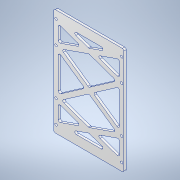
# Autodesk Inventor part: 関節2_上板
Saved by Autodesk Inventor 2021 (Build 250183000, 183)
## iProperties
Created: 2022-02-02
Part Number: 関節2_上板
Material: アルミニウム 6061
Document SubType Name: Modeling
Designer: hirohumi
Density: 2.7 g/cm^3
Appearance: アルミニウム - フラット
Mass: 103.807 g
Surface Area: 272.646 cm^2
Volume: 38.447 cm^3
Author: hirohumi
Autodesk Inventor part; units mm, degrees
ref_plane "YZ Plane" through (0, 0, 0) normal (1, 0, 0) x (0, 1, 0)
ref_plane "XZ Plane" through (0, 0, 0) normal (0, 1, 0) x (-1, 0, 0)
ref_plane "XY Plane" through (0, 0, 0) normal (0, 0, 1) x (1, 0, 0)
sketch "スケッチ1" plane through (0, 0, 0) normal (0, 0, 1) x (1, 0, 0)
  line L0 (46, 70) -> (-46, 70)
  line L1 (-46, 70) -> (-46, -70)
  line L2 (-46, -70) -> (46, -70)
  line L3 (46, -70) -> (46, 70)
  line L4 (46, 70) -> (-46, -70) construction
  line L5 (-46, 70) -> (46, -70) construction
  circle A0 centre (-43, 60) radius 1.6
  circle A1 centre (-43, 30) radius 1.6
  circle A2 centre (-43, -30) radius 1.6
  circle A3 centre (-43, -60) radius 1.6
  circle A4 centre (43, 60) radius 1.6
  circle A5 centre (43, 30) radius 1.6
  circle A6 centre (43, -30) radius 1.6
  circle A7 centre (43, -60) radius 1.6
  point P0 (0, 0)
  dimension "d0" = 92
  dimension "d1" = 140
  dimension "d2" = 3.2
  dimension "d3" = 3.2
  dimension "d4" = 3.2
  dimension "d5" = 3.2
  dimension "d6" = 120
  dimension "d7" = 10
  dimension "d8" = 30
  dimension "d9" = 30
  dimension "d10" = 3.2
  dimension "d11" = 3.2
  dimension "d12" = 3.2
  dimension "d13" = 3.2
  dimension "d14" = 120
  dimension "d15" = 30
  dimension "d16" = 30
  dimension "d17" = 3
  dimension "d18" = 3
  dimension "d19" = 60
  constraints: 12 end point, 8 centre point, 6 vertical alignment, 2 midpoint, 2 parallel, 1 horizontal, 1 perpendicular
  measures "d0" distance of L2.end L1.end
  measures "d1" distance of L1.end L0.end
  measures "d2" diameter of A0
  measures "d3" diameter of A1
  measures "d4" diameter of A2
  measures "d5" diameter of A3
  measures "d6" distance of A3.centre A0.centre
  measures "d7" distance from line of L0 A0.centre
  measures "d8" distance of A1.centre A0.centre
  measures "d9" distance of A3.centre A2.centre
  measures "d10" diameter of A4
  measures "d11" diameter of A5
  measures "d12" diameter of A6
  measures "d13" diameter of A7
  measures "d14" distance of A7.centre A4.centre
  measures "d15" distance of A5.centre A4.centre
  measures "d16" distance of A7.centre A6.centre
  measures "d17" distance from line of L1 A1.centre
  measures "d18" distance from line of L3 A5.centre
  measures "d19" vertical distance of point (0, 0) A4.centre
extrude "押し出し1" add sketch "スケッチ1" along normal blind 3
fillet "フィレット1" radius 2 4 edges at (-46, 70, 1.5) (46, 70, 1.5) (-46, -70, 1.5) (46, -70, 1.5)
sketch "スケッチ2" plane through (0, 0, 3) normal (0, 0, 1) x (1, 0, 0)
  circle A0 centre (-43, 60) radius 1.6 projected
  circle A1 centre (43, 30) radius 1.6 projected
  line L0 (-43, 60) -> (43, 30) construction
  circle A2 centre (-43, 30) radius 1.6 projected
  circle A3 centre (43, -30) radius 1.6 projected
  line L1 (-43, 30) -> (43, -30) construction
  circle A4 centre (-43, -60) radius 1.6 projected
  line L2 (43, -30) -> (-43, -60) construction
  circle A5 centre (43, -60) radius 1.6 projected
  line L3 (-43, -60) -> (43, -60) construction
  circle A6 centre (-43, -30) radius 1.6 projected
  line L4 (43, -60) -> (-43, -30) construction
  line L5 (-43, -30) -> (43, 30) construction
  circle A7 centre (43, 60) radius 1.6 projected
  line L6 (-43, 60) -> (43, 60) construction
  line L7 (43, 60) -> (-43, 30) construction
  line L8 (-43, 60) -> (-43, -60) construction
  line L9 (43, 60) -> (43, -60) construction
  line L10 (-40, 55.7762) -> (-40, 34.2238)
  line L11 (-40, 34.2238) -> (-9.1082, 45)
  line L12 (-9.1082, 45) -> (-40, 55.7762)
  line L13 (9.1082, 45) -> (40, 34.2238)
  line L14 (40, 34.2238) -> (40, 55.7762)
  line L15 (40, 55.7762) -> (9.1082, 45)
  line L16 (-28.1584, 58) -> (0, 48.1773)
  line L17 (0, 48.1773) -> (28.1584, 58)
  line L18 (28.1584, 58) -> (-28.1584, 58)
  line L19 (-36.4685, 29.1011) -> (0, 41.8227)
  line L20 (0, 41.8227) -> (36.4685, 29.1011)
  line L21 (36.4685, 29.1011) -> (0, 3.658)
  line L22 (0, 3.658) -> (-36.4685, 29.1011)
  line L23 (-40, 24.249) -> (-40, -24.249)
  line L24 (-40, -24.249) -> (-5.2431, 0)
  line L25 (-5.2431, 0) -> (-40, 24.249)
  line L26 (5.2431, 0) -> (40, -24.249)
  line L27 (40, -24.249) -> (40, 24.249)
  line L28 (5.2431, 0) -> (40, 24.249)
  line L29 (-36.4685, -29.1011) -> (0, -41.8227)
  line L30 (0, -41.8227) -> (36.4685, -29.1011)
  line L31 (36.4685, -29.1011) -> (0, -3.658)
  line L32 (0, -3.658) -> (-36.4685, -29.1011)
  line L33 (-40, -34.2238) -> (-40, -55.7762)
  line L34 (-40, -55.7762) -> (-9.1082, -45)
  line L35 (-9.1082, -45) -> (-40, -34.2238)
  line L36 (9.1082, -45) -> (40, -55.7762)
  line L37 (40, -55.7762) -> (40, -34.2238)
  line L38 (40, -34.2238) -> (9.1082, -45)
  line L39 (0, -48.1773) -> (-28.1584, -58)
  line L40 (-28.1584, -58) -> (28.1584, -58)
  line L41 (28.1584, -58) -> (0, -48.1773)
  point P0 (0, 0)
  dimension "d23" = 2
  dimension "d24" = 3
  dimension "d25" = 3
  dimension "d26" = 3
  dimension "d27" = 3
  dimension "d28" = 3
  dimension "d29" = 3
  dimension "d30" = 3
  dimension "d31" = 3
  dimension "d32" = 3
  dimension "d33" = 3
  dimension "d34" = 3
  dimension "d35" = 3
  dimension "d36" = 3
  dimension "d37" = 3
  dimension "d38" = 3
  dimension "d39" = 3
  dimension "d40" = 3
  dimension "d41" = 3
  dimension "d42" = 3
  dimension "d43" = 3
  dimension "d44" = 3
  dimension "d45" = 3
  dimension "d46" = 3
  dimension "d47" = 3
  dimension "d48" = 3
  dimension "d49" = 3
  dimension "d50" = 3
  dimension "d51" = 3
  dimension "d52" = 2
  constraints: 84 end point, 33 parallel, 2 point on line, 1 collinear, 1 horizontal, 1 vertical
  measures "d23" distance between parallel lines of L6 L18
  measures "d24" distance between parallel lines of L0 L16
  measures "d25" distance between parallel lines of L7 L17
  measures "d26" distance between parallel lines of L0 L12
  measures "d27" distance between parallel lines of L7 L15
  measures "d28" distance between parallel lines of L9 L14
  measures "d29" distance between parallel lines of L8 L10
  measures "d30" distance between parallel lines of L7 L19
  measures "d31" distance between parallel lines of L0 L20
  measures "d32" distance between parallel lines of L5 L21
  measures "d33" distance between parallel lines of L1 L22
  measures "d34" distance between parallel lines of L1 L25
  measures "d35" distance between parallel lines of L5 L24
  measures "d36" distance between parallel lines of L8 L23
  measures "d37" distance between parallel lines of L5 L28
  measures "d38" distance between parallel lines of L1 L26
  measures "d39" distance between parallel lines of L9 L27
  measures "d40" distance between parallel lines of L1 L31
  measures "d41" distance between parallel lines of L5 L32
  measures "d42" distance between parallel lines of L4 L29
  measures "d43" distance between parallel lines of L2 L30
  measures "d44" distance between parallel lines of L4 L35
  measures "d45" distance between parallel lines of L8 L33
  measures "d46" distance between parallel lines of L2 L34
  measures "d47" distance between parallel lines of L2 L38
  measures "d48" distance between parallel lines of L4 L36
  measures "d49" distance between parallel lines of L9 L37
  measures "d50" distance between parallel lines of L4 L41
  measures "d51" distance between parallel lines of L2 L39
  measures "d52" distance between parallel lines of L3 L40
extrude "押し出し2" cut sketch "スケッチ2" against normal through all contours L12 L11 L10 | L15 L14 L13 | L18 L17 L16 | L19 L20 L21 L22 | L25 L24 L23 | L28 L27 L26 | L32 L31 L30 L29 | L35 L34 L33 | L38 L37 L36 | L41 L40 L39
fillet "フィレット2" radius 2 32 edges at (-40, -55.7762, 1.5) (-40, -34.2238, 1.5) (-9.1082, -45, 1.5) (-28.1584, -58, 1.5) (0, -48.1773, 1.5) (28.1584, -58, 1.5) (40, -55.7762, 1.5) (9.1082, -45, 1.5) (40, -34.2238, 1.5) (0, -41.8227, 1.5) (-36.4685, -29.1011, 1.5) (36.4685, -29.1011, 1.5) (0, -3.658, 1.5) (-40, -24.249, 1.5) (-40, 24.249, 1.5) (-5.2431, 0, 1.5) (-40, 34.2238, 1.5) (-40, 55.7762, 1.5) (-9.1082, 45, 1.5) (0, 48.1773, 1.5) (-28.1584, 58, 1.5) (28.1584, 58, 1.5) (0, 3.658, 1.5) (-36.4685, 29.1011, 1.5) (36.4685, 29.1011, 1.5) (0, 41.8227, 1.5) (40, -24.249, 1.5) (5.2431, 0, 1.5) (40, 24.249, 1.5) (40, 34.2238, 1.5) (9.1082, 45, 1.5) (40, 55.7762, 1.5)
